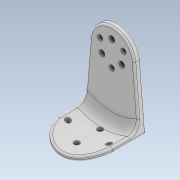
# Autodesk Inventor part: shank_thigh_connector
Saved by Autodesk Inventor 2020 (Build 240168000, 168)
## iProperties
Created: 2021-01-06
Part Number: shank_thigh_connector
Material: Generic
Document SubType Name: Modeling
Designer: DELL
Density: 1 g/cm^3
Appearance: Clear - Blue
Author: DELL
Autodesk Inventor part; units mm, degrees
ref_plane "YZ Plane" through (0, 0, 0) normal (1, 0, 0) x (0, 1, 0)
ref_plane "XZ Plane" through (0, 0, 0) normal (0, 1, 0) x (-1, 0, 0)
ref_plane "XY Plane" through (0, 0, 0) normal (0, 0, 1) x (1, 0, 0)
sketch "Sketch1" plane through (0, 0, 0) normal (0, 0, 1) x (1, 0, 0)
  circle A0 centre (0, 0) radius 19
  line L0 (-18.933615, 1.586891) -> (-23.333333, -50.907323)
  line L1 (18.933615, 1.586891) -> (23.333333, -50.907323)
  line L2 (9.959292, -5.75) -> (0, 0) construction
  circle A1 centre (8.413437, -4.8575) radius 2.5
  line L3 (0, 0) -> (9.959292, 5.75) construction
  line L4 (0, 0) -> (-9.959292, -5.75) construction
  circle A2 centre (-8.413437, -4.8575) radius 2.5
  circle A3 centre (0, 0) radius 9.715 construction
  circle A4 centre (0, 0) radius 11.5 construction
  circle A5 centre (0, 9.715) radius 2.5
  line L5 (0, 0) -> (-9.959292, 5.75) construction
  line L6 (11.5, 0) -> (-11.5, 0) construction
  circle A6 centre (-9.959292, 5.75) radius 4
  circle A7 centre (-9.959292, 5.75) radius 2.25
  line L7 (0, -48.572131) -> (0, 22.5) construction
  circle A8 centre (0, -11.5) radius 2.25
  circle A9 centre (0, -11.5) radius 4
  circle A10 centre (9.959292, 5.75) radius 4
  circle A11 centre (9.959292, 5.75) radius 2.25
  arc A12 (-22.97639, -46.648532) -> (22.97639, -46.648532) centre (0, 0) ccw
  arc A13 (-23.333333, -50.907323) -> (23.333333, -50.907323) centre (0, 0) ccw
  line L8 (0, 0) -> (-23.333333, -50.907323) construction
  point P0 (0, 11.468562)
  point P1 (0, 11.468562)
  point P2 (11.5, 0)
  point P3 (-11.5, 0)
  dimension "d18" = 23
  dimension "d0" = 38
  dimension "d17" = 19.43
  dimension "d19" = 30
  dimension "d20" = 30
  dimension "d21" = 4.5
  dimension "d22" = 8
  dimension "d23" = 5
  dimension "d24" = 104
  dimension "d25" = 112
  dimension "d58" = 24.6243
  constraints: 16 end point, 13 centre point, 10 coincident, 9 point on circle, 8 point on line, 6 equal radius, 2 tangent, 1 vertical, 17 other
  measures "d0" diameter of A0
  measures "d17" diameter of A3
  measures "d19" angle to the sketch x axis of L5
  measures "d20" angle to the sketch x axis of L4
  measures "d21" diameter of A11
  measures "d22" diameter of A10
  measures "d23" diameter of A5
  measures "d24" diameter of A12
  measures "d25" diameter of A13
  measures "d58" angle of L7 L8
sketch "Sketch1 outline for Extrusion1" plane through (0, 0, 0) normal (0, 0, 1) x (1, 0, 0)
  arc A0 (18.933615, 1.586891) -> (-18.933615, 1.586891) centre (0, 0) ccw
  line L0 (23.333333, -50.907323) -> (18.933615, 1.586891)
  line L1 (-18.933615, 1.586891) -> (-23.333333, -50.907323)
  arc A1 (-23.333333, -50.907323) -> (23.333333, -50.907323) centre (0, 0) ccw
  circle A2 centre (0, -11.5) radius 2.25
  circle A3 centre (-9.959292, 5.75) radius 2.25
  circle A4 centre (9.959292, 5.75) radius 2.25
extrude "Extrusion1" add sketch "Sketch1 outline for Extrusion1" along normal blind 6
sketch "Sketch1 outline for Extrusion2" plane through (0, 0, 0) normal (0, 0, 1) x (1, 0, 0)
  circle A0 centre (0, -11.5) radius 4
  circle A1 centre (0, -11.5) radius 2.25
  circle A2 centre (-9.959292, 5.75) radius 4
  circle A3 centre (-9.959292, 5.75) radius 2.25
  circle A4 centre (9.959292, 5.75) radius 4
extrude "Extrusion2" cut sketch "Sketch1 outline for Extrusion2" along normal blind 3
sketch "Sketch1 outline for Extrusion3" plane through (0, 0, 0) normal (0, 0, 1) x (1, 0, 0)
  circle A0 centre (0, 9.715) radius 2.5
  circle A1 centre (-8.413437, -4.8575) radius 2.5
  circle A2 centre (8.413437, -4.8575) radius 2.5
extrude "Extrusion3" cut sketch "Sketch1 outline for Extrusion3" along normal through all
sketch "Sketch1 outline for Extrusion4" plane through (0, 0, 0) normal (0, 0, 1) x (1, 0, 0)
  arc A0 (-23.333333, -50.907323) -> (23.333333, -50.907323) centre (0, 0) ccw
  line L0 (-22.97639, -46.648532) -> (-23.333333, -50.907323)
  arc A1 (22.97639, -46.648532) -> (-22.97639, -46.648532) centre (0, 0) cw
  line L1 (23.333333, -50.907323) -> (22.97639, -46.648532)
extrude "Extrusion4" add sketch "Sketch1 outline for Extrusion4" along normal blind 47.5 from surface at 6
sketch "Sketch3" plane through (0, 0, 0) normal (0, 1, 0) x (-1, 0, 0)
  circle A0 centre (0, 16) radius 2.25
  circle A1 centre (0, 36) radius 2.25
  circle A2 centre (0, 36) radius 1.5
  circle A3 centre (0, 16) radius 1.5
  line L0 (-23.333333, 26) -> (24.035112, 26) construction
  line L1 (0, 10.215554) -> (0, 41.784446) construction
  circle A4 centre (-17.5, 26) radius 1.5
  circle A5 centre (-17.5, 26) radius 2.25
  circle A6 centre (17.5, 26) radius 1.5
  circle A7 centre (17.5, 26) radius 2.25
  circle A8 centre (0, 26) radius 6
  circle A9 centre (0, 26) radius 23.333333
  line L2 (22.97639, 53.5) -> (-22.97639, 53.5)
  line L3 (23.333333, 26) -> (23.333333, 53.5)
  line L4 (23.333333, 53.5) -> (-23.333333, 53.5)
  line L5 (-23.333333, 53.5) -> (-23.333333, 26)
  line L6 (23.333333, 0) -> (23.333333, 53.5)
  line L7 (-23.333333, 0) -> (-23.333333, 53.5)
  point P0 (0, 0)
  point P1 (-23.333333, 26)
  dimension "d42" = 4.5
  dimension "d43" = 3
  dimension "d44" = 20
  dimension "d45" = 35
  dimension "d46" = 12
  dimension "d60" = 27.5
  constraints: 10 end point, 9 centre point, 6 equal radius, 5 coincident, 4 point on line, 3 collinear, 3 vertical, 2 perpendicular, 2 symmetric about line, 1 horizontal, 1 midpoint, 3 other
  measures "d42" diameter of A1
  measures "d43" diameter of A2
  measures "d44" distance of A1.centre A0.centre
  measures "d45" distance of A6.centre A4.centre
  measures "d46" diameter of A8
  measures "d60" distance between parallel lines of L2 L0
sketch "Sketch3 outline for Extrusion8" plane through (0, 0, 0) normal (0, 1, 0) x (-1, 0, 0)
  circle A0 centre (0, 16) radius 1.5
  line L0 (-23.333333, 53.5) -> (-23.333333, 26)
  arc A1 (-23.333333, 26) -> (23.333333, 26) centre (0, 26) cw
  line L1 (23.333333, 26) -> (23.333333, 53.5)
  line L2 (23.333333, 53.5) -> (-23.333333, 53.5)
  circle A2 centre (0, 36) radius 1.5
  circle A3 centre (-17.5, 26) radius 1.5
  circle A4 centre (17.5, 26) radius 1.5
extrude "Extrusion8" cut sketch "Sketch3 outline for Extrusion8" against normal through all
sketch "Sketch3 outline for Extrusion13" plane through (0, 0, 0) normal (0, 1, 0) x (-1, 0, 0)
  circle A0 centre (0, 16) radius 2.25
  circle A1 centre (0, 36) radius 2.25
extrude "Extrusion13" cut sketch "Sketch3 outline for Extrusion13" against normal blind 54
sketch "Sketch3 outline for Extrusion14" plane through (0, 0, 0) normal (0, 1, 0) x (-1, 0, 0)
  circle A0 centre (-17.5, 26) radius 2.25
  circle A1 centre (17.5, 26) radius 2.25
extrude "Extrusion14" cut sketch "Sketch3 outline for Extrusion14" against normal blind 50
fillet "Fillet1" radius 8 1 edges at (0, -52, 6)
fillet "Fillet2" radius 1.5 15 edges at (0, -56, 0) (23.3333, -50.9073, 13) (-23.3333, -50.9073, 13) (-21.1335, -24.6602, 0) (21.1335, -24.6602, 0) (0, 19, 0) (-20.5909, -18.1869, 6) (-22.7531, -43.9844, 8.2105) (-22.9764, -46.6485, 22.0329) (20.5909, -18.1869, 6) (22.7531, -43.9844, 8.2105) (22.9764, -46.6485, 22.0329) (0, 19, 6) (-0.0001, -52, 49.3333) (0.0003, -56, 49.3333)
body "Solid1"
